Autodesk Inventor part; units mm, degrees
(part 2 of 2)
sketch "Triangle Hole Template x16_1" plane through (0, 0, 0) normal (0, 0, 1) x (1, 0, 0)
  line L0 (-16.6681, -28.8484) -> (-50.0011, -28.8484) construction
  line L1 (-50.0011, -28.8484) -> (-33.3346, 0.0188) construction
  line L2 (-33.3346, 0.0188) -> (-16.6681, -28.8484) construction
  line L3 (-17.5341, -28.3484) -> (-49.1351, -28.3484) construction
  line L4 (-33.3346, -28.8484) -> (-33.3346, -29.3484) construction
  line L5 (-18.5734, -27.7484) -> (-19.2662, -27.3484) construction
  line L6 (-49.1351, -28.3484) -> (-33.3346, -0.9812) construction
  line L7 (-33.3346, -0.9812) -> (-17.5341, -28.3484) construction
  line L8 (-33.3346, -28.3484) -> (-33.3346, -28.8484) construction
  line L9 (-41.2348, -14.6648) -> (-41.6679, -14.4148) construction
  line L10 (-25.4344, -14.6648) -> (-25.0014, -14.4148) construction
  arc A0 (-48.0959, -26.5484) -> (-47.0566, -28.3484) centre (-47.0566, -27.1484) ccw
  arc A1 (-32.2954, -2.7812) -> (-34.3738, -2.7812) centre (-33.3346, -3.3812) ccw
  arc A2 (-19.6126, -28.3484) -> (-18.5734, -26.5484) centre (-19.6126, -27.1484) ccw
  line L11 (-19.6126, -28.3484) -> (-47.0566, -28.3484)
  line L12 (-48.0959, -26.5484) -> (-34.3738, -2.7812)
  line L13 (-32.2954, -2.7812) -> (-18.5734, -26.5484)
  circle A3 centre (-18.227, -27.9484) radius 0.4 construction
  line L14 (-18.5734, -27.7484) -> (-17.8805, -28.1484) construction
  circle A4 centre (-16.6681, -28.8484) radius 3 construction
  line L15 (-49.9979, -28.8484) -> (-16.6649, -28.8484) construction
  line L16 (-16.6649, -28.8484) -> (-33.3314, -57.7156) construction
  line L17 (-33.3314, -57.7156) -> (-49.9979, -28.8484) construction
  line L18 (-49.1319, -29.3484) -> (-17.5309, -29.3484) construction
  line L19 (-33.3314, -28.8484) -> (-33.3314, -28.3484) construction
  line L20 (-48.0926, -29.9484) -> (-47.3998, -30.3484) construction
  line L21 (-17.5309, -29.3484) -> (-33.3314, -56.7156) construction
  line L22 (-33.3314, -56.7156) -> (-49.1319, -29.3484) construction
  line L23 (-33.3314, -29.3484) -> (-33.3314, -28.8484) construction
  line L24 (-25.4312, -43.032) -> (-24.9981, -43.282) construction
  line L25 (-41.2316, -43.032) -> (-41.6646, -43.282) construction
  arc A5 (-18.5701, -31.1484) -> (-19.6094, -29.3484) centre (-19.6094, -30.5484) ccw
  arc A6 (-34.3706, -54.9156) -> (-32.2922, -54.9156) centre (-33.3314, -54.3156) ccw
  arc A7 (-47.0534, -29.3484) -> (-48.0926, -31.1484) centre (-47.0534, -30.5484) ccw
  line L26 (-47.0534, -29.3484) -> (-19.6094, -29.3484)
  line L27 (-18.5701, -31.1484) -> (-32.2922, -54.9156)
  line L28 (-34.3706, -54.9156) -> (-48.0926, -31.1484)
  circle A8 centre (-48.439, -29.7484) radius 0.4 construction
  line L29 (-48.0926, -29.9484) -> (-48.7855, -29.5484) construction
  circle A9 centre (-49.9979, -28.8484) radius 3 construction
  line L30 (-66.6676, 0.0188) -> (-33.3346, 0.0188) construction
  line L31 (-33.3346, 0.0188) -> (-50.0011, -28.8484) construction
  line L32 (-50.0011, -28.8484) -> (-66.6676, 0.0188) construction
  line L33 (-65.8016, -0.4812) -> (-34.2006, -0.4812) construction
  line L34 (-50.0011, 0.0188) -> (-50.0011, 0.5188) construction
  line L35 (-64.7624, -1.0812) -> (-64.0695, -1.4812) construction
  line L36 (-34.2006, -0.4812) -> (-50.0011, -27.8484) construction
  line L37 (-50.0011, -27.8484) -> (-65.8016, -0.4812) construction
  line L38 (-50.0011, -0.4812) -> (-50.0011, 0.0188) construction
  line L39 (-42.1009, -14.1648) -> (-41.6679, -14.4148) construction
  line L40 (-57.9013, -14.1648) -> (-58.3344, -14.4148) construction
  arc A10 (-35.2399, -2.2812) -> (-36.2791, -0.4812) centre (-36.2791, -1.6812) ccw
  arc A11 (-51.0403, -26.0484) -> (-48.9619, -26.0484) centre (-50.0011, -25.4484) ccw
  arc A12 (-63.7231, -0.4812) -> (-64.7624, -2.2812) centre (-63.7231, -1.6812) ccw
  line L41 (-63.7231, -0.4812) -> (-36.2791, -0.4812)
  line L42 (-35.2399, -2.2812) -> (-48.9619, -26.0484)
  line L43 (-51.0403, -26.0484) -> (-64.7624, -2.2812)
  circle A13 centre (-65.1088, -0.8812) radius 0.4 construction
  line L44 (-64.7624, -1.0812) -> (-65.4552, -0.6812) construction
  circle A14 centre (-66.6676, 0.0188) radius 3 construction
  line L45 (-33.3314, 0.0188) -> (0.0016, 0.0188) construction
  line L46 (0.0016, 0.0188) -> (-16.6649, -28.8484) construction
  line L47 (-16.6649, -28.8484) -> (-33.3314, 0.0188) construction
  line L48 (-32.4654, -0.4812) -> (-0.8644, -0.4812) construction
  line L49 (-16.6649, 0.0188) -> (-16.6649, 0.5188) construction
  line L50 (-31.4261, -1.0812) -> (-30.7333, -1.4812) construction
  line L51 (-0.8644, -0.4812) -> (-16.6649, -27.8484) construction
  line L52 (-16.6649, -27.8484) -> (-32.4654, -0.4812) construction
  line L53 (-16.6649, -0.4812) -> (-16.6649, 0.0188) construction
  line L54 (-8.7647, -14.1648) -> (-8.3316, -14.4148) construction
  line L55 (-24.5651, -14.1648) -> (-24.9981, -14.4148) construction
  arc A15 (-1.9036, -2.2812) -> (-2.9429, -0.4812) centre (-2.9429, -1.6812) ccw
  arc A16 (-17.7041, -26.0484) -> (-15.6257, -26.0484) centre (-16.6649, -25.4484) ccw
  arc A17 (-30.3869, -0.4812) -> (-31.4261, -2.2812) centre (-30.3869, -1.6812) ccw
  line L56 (-30.3869, -0.4812) -> (-2.9429, -0.4812)
  line L57 (-1.9036, -2.2812) -> (-15.6257, -26.0484)
  line L58 (-17.7041, -26.0484) -> (-31.4261, -2.2812)
  circle A18 centre (-31.7725, -0.8812) radius 0.4 construction
  line L59 (-31.4261, -1.0812) -> (-32.119, -0.6812) construction
  circle A19 centre (-33.3314, 0.0188) radius 3 construction
  line L60 (-83.317, -28.8188) -> (-49.984, -28.8188) construction
  line L61 (-49.984, -28.8188) -> (-66.6505, -57.686) construction
  line L62 (-66.6505, -57.686) -> (-83.317, -28.8188) construction
  line L63 (-82.451, -29.3188) -> (-50.85, -29.3188) construction
  line L64 (-66.6505, -28.8188) -> (-66.6505, -28.3188) construction
  line L65 (-81.4117, -29.9188) -> (-80.7189, -30.3188) construction
  line L66 (-50.85, -29.3188) -> (-66.6505, -56.686) construction
  line L67 (-66.6505, -56.686) -> (-82.451, -29.3188) construction
  line L68 (-66.6505, -29.3188) -> (-66.6505, -28.8188) construction
  line L69 (-58.7503, -43.0024) -> (-58.3173, -43.2524) construction
  line L70 (-74.5507, -43.0024) -> (-74.9838, -43.2524) construction
  arc A20 (-51.8893, -31.1188) -> (-52.9285, -29.3188) centre (-52.9285, -30.5188) ccw
  arc A21 (-67.6897, -54.886) -> (-65.6113, -54.886) centre (-66.6505, -54.286) ccw
  arc A22 (-80.3725, -29.3188) -> (-81.4117, -31.1188) centre (-80.3725, -30.5188) ccw
  line L71 (-80.3725, -29.3188) -> (-52.9285, -29.3188)
  line L72 (-51.8893, -31.1188) -> (-65.6113, -54.886)
  line L73 (-67.6897, -54.886) -> (-81.4117, -31.1188)
  circle A23 centre (-81.7582, -29.7188) radius 0.4 construction
  line L74 (-81.4117, -29.9188) -> (-82.1046, -29.5188) construction
  circle A24 centre (-83.317, -28.8188) radius 3 construction
  line L75 (-99.9974, 0.0188) -> (-66.6644, 0.0188) construction
  line L76 (-66.6644, 0.0188) -> (-83.3309, -28.8484) construction
  line L77 (-83.3309, -28.8484) -> (-99.9974, 0.0188) construction
  line L78 (-99.1314, -0.4812) -> (-67.5304, -0.4812) construction
  line L79 (-83.3309, 0.0188) -> (-83.3309, 0.5188) construction
  line L80 (-98.0921, -1.0812) -> (-97.3993, -1.4812) construction
  line L81 (-67.5304, -0.4812) -> (-83.3309, -27.8484) construction
  line L82 (-83.3309, -27.8484) -> (-99.1314, -0.4812) construction
  line L83 (-83.3309, -0.4812) -> (-83.3309, 0.0188) construction
  line L84 (-75.4307, -14.1648) -> (-74.9976, -14.4148) construction
  line L85 (-91.2311, -14.1648) -> (-91.6641, -14.4148) construction
  arc A25 (-68.5696, -2.2812) -> (-69.6089, -0.4812) centre (-69.6089, -1.6812) ccw
  arc A26 (-84.3701, -26.0484) -> (-82.2917, -26.0484) centre (-83.3309, -25.4484) ccw
  arc A27 (-97.0529, -0.4812) -> (-98.0921, -2.2812) centre (-97.0529, -1.6812) ccw
  line L86 (-97.0529, -0.4812) -> (-69.6089, -0.4812)
  line L87 (-68.5696, -2.2812) -> (-82.2917, -26.0484)
  line L88 (-84.3701, -26.0484) -> (-98.0921, -2.2812)
  circle A28 centre (-98.4385, -0.8812) radius 0.4 construction
  line L89 (-98.0921, -1.0812) -> (-98.785, -0.6812) construction
  circle A29 centre (-99.9974, 0.0188) radius 3 construction
  line L90 (-133.3304, -0.008) -> (-99.9974, -0.008) construction
  line L91 (-99.9974, -0.008) -> (-116.6639, -28.8752) construction
  line L92 (-116.6639, -28.8752) -> (-133.3304, -0.008) construction
  line L93 (-132.4644, -0.508) -> (-100.8634, -0.508) construction
  line L94 (-116.6639, -0.008) -> (-116.6639, 0.492) construction
  line L95 (-131.4251, -1.108) -> (-130.7323, -1.508) construction
  line L96 (-100.8634, -0.508) -> (-116.6639, -27.8752) construction
  line L97 (-116.6639, -27.8752) -> (-132.4644, -0.508) construction
  line L98 (-116.6639, -0.508) -> (-116.6639, -0.008) construction
  line L99 (-108.7637, -14.1916) -> (-108.3306, -14.4416) construction
  line L100 (-124.5641, -14.1916) -> (-124.9971, -14.4416) construction
  arc A30 (-101.9026, -2.308) -> (-102.9419, -0.508) centre (-102.9419, -1.708) ccw
  arc A31 (-117.7031, -26.0752) -> (-115.6247, -26.0752) centre (-116.6639, -25.4752) ccw
  arc A32 (-130.3859, -0.508) -> (-131.4251, -2.308) centre (-130.3859, -1.708) ccw
  line L101 (-130.3859, -0.508) -> (-102.9419, -0.508)
  line L102 (-101.9026, -2.308) -> (-115.6247, -26.0752)
  line L103 (-117.7031, -26.0752) -> (-131.4251, -2.308)
  circle A33 centre (-131.7715, -0.908) radius 0.4 construction
  line L104 (-131.4251, -1.108) -> (-132.118, -0.708) construction
  circle A34 centre (-133.3304, -0.008) radius 3 construction
  line L105 (-116.6671, -28.8484) -> (-83.3341, -28.8484) construction
  line L106 (-83.3341, -28.8484) -> (-100.0006, -57.7156) construction
  line L107 (-100.0006, -57.7156) -> (-116.6671, -28.8484) construction
  line L108 (-115.8011, -29.3484) -> (-84.2001, -29.3484) construction
  line L109 (-100.0006, -28.8484) -> (-100.0006, -28.3484) construction
  line L110 (-114.7619, -29.9484) -> (-114.069, -30.3484) construction
  line L111 (-84.2001, -29.3484) -> (-100.0006, -56.7156) construction
  line L112 (-100.0006, -56.7156) -> (-115.8011, -29.3484) construction
  line L113 (-100.0006, -29.3484) -> (-100.0006, -28.8484) construction
  line L114 (-92.1004, -43.032) -> (-91.6674, -43.282) construction
  line L115 (-107.9008, -43.032) -> (-108.3339, -43.282) construction
  arc A35 (-85.2394, -31.1484) -> (-86.2786, -29.3484) centre (-86.2786, -30.5484) ccw
  arc A36 (-101.0398, -54.9156) -> (-98.9614, -54.9156) centre (-100.0006, -54.3156) ccw
  arc A37 (-113.7226, -29.3484) -> (-114.7619, -31.1484) centre (-113.7226, -30.5484) ccw
  line L116 (-113.7226, -29.3484) -> (-86.2786, -29.3484)
  line L117 (-85.2394, -31.1484) -> (-98.9614, -54.9156)
  line L118 (-101.0398, -54.9156) -> (-114.7619, -31.1484)
  circle A38 centre (-115.1083, -29.7484) radius 0.4 construction
  line L119 (-114.7619, -29.9484) -> (-115.4547, -29.5484) construction
  circle A39 centre (-116.6671, -28.8484) radius 3 construction
  line L120 (-99.9974, -57.7156) -> (-66.6644, -57.7156) construction
  line L121 (-66.6644, -57.7156) -> (-83.3309, -86.5829) construction
  line L122 (-83.3309, -86.5829) -> (-99.9974, -57.7156) construction
  line L123 (-99.1314, -58.2156) -> (-67.5304, -58.2156) construction
  line L124 (-83.3309, -57.7156) -> (-83.3309, -57.2156) construction
  line L125 (-98.0921, -58.8156) -> (-97.3993, -59.2156) construction
  line L126 (-67.5304, -58.2156) -> (-83.3309, -85.5829) construction
  line L127 (-83.3309, -85.5829) -> (-99.1314, -58.2156) construction
  line L128 (-83.3309, -58.2156) -> (-83.3309, -57.7156) construction
  line L129 (-75.4307, -71.8992) -> (-74.9976, -72.1492) construction
  line L130 (-91.2311, -71.8992) -> (-91.6641, -72.1492) construction
  arc A40 (-68.5696, -60.0156) -> (-69.6089, -58.2156) centre (-69.6089, -59.4156) ccw
  arc A41 (-84.3701, -83.7829) -> (-82.2917, -83.7829) centre (-83.3309, -83.1829) ccw
  arc A42 (-97.0529, -58.2156) -> (-98.0921, -60.0156) centre (-97.0529, -59.4156) ccw
  line L131 (-97.0529, -58.2156) -> (-69.6089, -58.2156)
  line L132 (-68.5696, -60.0156) -> (-82.2917, -83.7829)
  line L133 (-84.3701, -83.7829) -> (-98.0921, -60.0156)
  circle A43 centre (-98.4385, -58.6156) radius 0.4 construction
  line L134 (-98.0921, -58.8156) -> (-98.785, -58.4156) construction
  circle A44 centre (-99.9974, -57.7156) radius 3 construction
  line L135 (-83.3309, -86.5829) -> (-49.9979, -86.5829) construction
  line L136 (-49.9979, -86.5829) -> (-66.6644, -115.4501) construction
  line L137 (-66.6644, -115.4501) -> (-83.3309, -86.5829) construction
  line L138 (-82.4649, -87.0829) -> (-50.8639, -87.0829) construction
  line L139 (-66.6644, -86.5829) -> (-66.6644, -86.0829) construction
  line L140 (-81.4256, -87.6829) -> (-80.7328, -88.0829) construction
  line L141 (-50.8639, -87.0829) -> (-66.6644, -114.4501) construction
  line L142 (-66.6644, -114.4501) -> (-82.4649, -87.0829) construction
  line L143 (-66.6644, -87.0829) -> (-66.6644, -86.5829) construction
  line L144 (-58.7642, -100.7665) -> (-58.3311, -101.0165) construction
  line L145 (-74.5646, -100.7665) -> (-74.9976, -101.0165) construction
  arc A45 (-51.9031, -88.8829) -> (-52.9424, -87.0829) centre (-52.9424, -88.2829) ccw
  arc A46 (-67.7036, -112.6501) -> (-65.6252, -112.6501) centre (-66.6644, -112.0501) ccw
  arc A47 (-80.3864, -87.0829) -> (-81.4256, -88.8829) centre (-80.3864, -88.2829) ccw
  line L146 (-80.3864, -87.0829) -> (-52.9424, -87.0829)
  line L147 (-51.9031, -88.8829) -> (-65.6252, -112.6501)
  line L148 (-67.7036, -112.6501) -> (-81.4256, -88.8829)
  circle A48 centre (-81.772, -87.4829) radius 0.4 construction
  line L149 (-81.4256, -87.6829) -> (-82.1185, -87.2829) construction
  circle A49 centre (-83.3309, -86.5829) radius 3 construction
  line L150 (-66.6676, -57.7533) -> (-33.3346, -57.7533) construction
  line L151 (-33.3346, -57.7533) -> (-50.0011, -86.6205) construction
  line L152 (-50.0011, -86.6205) -> (-66.6676, -57.7533) construction
  line L153 (-65.8016, -58.2533) -> (-34.2006, -58.2533) construction
  line L154 (-50.0011, -57.7533) -> (-50.0011, -57.2533) construction
  line L155 (-64.7624, -58.8533) -> (-64.0695, -59.2533) construction
  line L156 (-34.2006, -58.2533) -> (-50.0011, -85.6205) construction
  line L157 (-50.0011, -85.6205) -> (-65.8016, -58.2533) construction
  line L158 (-50.0011, -58.2533) -> (-50.0011, -57.7533) construction
  line L159 (-42.1009, -71.9369) -> (-41.6679, -72.1869) construction
  line L160 (-57.9013, -71.9369) -> (-58.3344, -72.1869) construction
  arc A50 (-35.2399, -60.0533) -> (-36.2791, -58.2533) centre (-36.2791, -59.4533) ccw
  arc A51 (-51.0403, -83.8205) -> (-48.9619, -83.8205) centre (-50.0011, -83.2205) ccw
  arc A52 (-63.7231, -58.2533) -> (-64.7624, -60.0533) centre (-63.7231, -59.4533) ccw
  line L161 (-63.7231, -58.2533) -> (-36.2791, -58.2533)
  line L162 (-35.2399, -60.0533) -> (-48.9619, -83.8205)
  line L163 (-51.0403, -83.8205) -> (-64.7624, -60.0533)
  circle A53 centre (-65.1088, -58.6533) radius 0.4 construction
  line L164 (-64.7624, -58.8533) -> (-65.4552, -58.4533) construction
  circle A54 centre (-66.6676, -57.7533) radius 3 construction
  line L165 (-50.0011, -86.6205) -> (-83.3341, -86.6205) construction
  line L166 (-83.3341, -86.6205) -> (-66.6676, -57.7533) construction
  line L167 (-66.6676, -57.7533) -> (-50.0011, -86.6205) construction
  line L168 (-50.8671, -86.1205) -> (-82.4681, -86.1205) construction
  line L169 (-66.6676, -86.6205) -> (-66.6676, -87.1205) construction
  line L170 (-51.9064, -85.5205) -> (-52.5992, -85.1205) construction
  line L171 (-82.4681, -86.1205) -> (-66.6676, -58.7533) construction
  line L172 (-66.6676, -58.7533) -> (-50.8671, -86.1205) construction
  line L173 (-66.6676, -86.1205) -> (-66.6676, -86.6205) construction
  line L174 (-74.5678, -72.4369) -> (-75.0009, -72.1869) construction
  line L175 (-58.7674, -72.4369) -> (-58.3344, -72.1869) construction
  arc A55 (-81.4289, -84.3205) -> (-80.3896, -86.1205) centre (-80.3896, -84.9205) ccw
  arc A56 (-65.6284, -60.5533) -> (-67.7068, -60.5533) centre (-66.6676, -61.1533) ccw
  arc A57 (-52.9456, -86.1205) -> (-51.9064, -84.3205) centre (-52.9456, -84.9205) ccw
  line L176 (-52.9456, -86.1205) -> (-80.3896, -86.1205)
  line L177 (-81.4289, -84.3205) -> (-67.7068, -60.5533)
  line L178 (-65.6284, -60.5533) -> (-51.9064, -84.3205)
  circle A58 centre (-51.56, -85.7205) radius 0.4 construction
  line L179 (-51.9064, -85.5205) -> (-51.2135, -85.9205) construction
  circle A59 centre (-50.0011, -86.6205) radius 3 construction
  line L180 (-33.3346, -57.7533) -> (-66.6676, -57.7533) construction
  line L181 (-66.6676, -57.7533) -> (-50.0011, -28.886) construction
  line L182 (-50.0011, -28.886) -> (-33.3346, -57.7533) construction
  line L183 (-34.2006, -57.2533) -> (-65.8016, -57.2533) construction
  line L184 (-50.0011, -57.7533) -> (-50.0011, -58.2533) construction
  line L185 (-35.2399, -56.6533) -> (-35.9327, -56.2533) construction
  line L186 (-65.8016, -57.2533) -> (-50.0011, -29.886) construction
  line L187 (-50.0011, -29.886) -> (-34.2006, -57.2533) construction
  line L188 (-50.0011, -57.2533) -> (-50.0011, -57.7533) construction
  line L189 (-57.9013, -43.5697) -> (-58.3344, -43.3197) construction
  line L190 (-42.1009, -43.5697) -> (-41.6679, -43.3197) construction
  arc A60 (-64.7624, -55.4533) -> (-63.7231, -57.2533) centre (-63.7231, -56.0533) ccw
  arc A61 (-48.9619, -31.686) -> (-51.0403, -31.686) centre (-50.0011, -32.286) ccw
  arc A62 (-36.2791, -57.2533) -> (-35.2399, -55.4533) centre (-36.2791, -56.0533) ccw
  line L191 (-36.2791, -57.2533) -> (-63.7231, -57.2533)
  line L192 (-64.7624, -55.4533) -> (-51.0403, -31.686)
  line L193 (-48.9619, -31.686) -> (-35.2399, -55.4533)
  circle A63 centre (-34.8935, -56.8533) radius 0.4 construction
  line L194 (-35.2399, -56.6533) -> (-34.547, -57.0533) construction
  circle A64 centre (-33.3346, -57.7533) radius 3 construction
  line L195 (-66.6676, -57.7156) -> (-100.0006, -57.7156) construction
  line L196 (-100.0006, -57.7156) -> (-83.3341, -28.8484) construction
  line L197 (-83.3341, -28.8484) -> (-66.6676, -57.7156) construction
  line L198 (-67.5336, -57.2156) -> (-99.1346, -57.2156) construction
  line L199 (-83.3341, -57.7156) -> (-83.3341, -58.2156) construction
  line L200 (-68.5729, -56.6156) -> (-69.2657, -56.2156) construction
  line L201 (-99.1346, -57.2156) -> (-83.3341, -29.8484) construction
  line L202 (-83.3341, -29.8484) -> (-67.5336, -57.2156) construction
  line L203 (-83.3341, -57.2156) -> (-83.3341, -57.7156) construction
  line L204 (-91.2343, -43.532) -> (-91.6674, -43.282) construction
  line L205 (-75.4339, -43.532) -> (-75.0009, -43.282) construction
  arc A65 (-98.0954, -55.4156) -> (-97.0561, -57.2156) centre (-97.0561, -56.0156) ccw
  arc A66 (-82.2949, -31.6484) -> (-84.3733, -31.6484) centre (-83.3341, -32.2484) ccw
  arc A67 (-69.6121, -57.2156) -> (-68.5729, -55.4156) centre (-69.6121, -56.0156) ccw
  line L206 (-69.6121, -57.2156) -> (-97.0561, -57.2156)
  line L207 (-98.0954, -55.4156) -> (-84.3733, -31.6484)
  line L208 (-82.2949, -31.6484) -> (-68.5729, -55.4156)
  circle A68 centre (-68.2265, -56.8156) radius 0.4 construction
  line L209 (-68.5729, -56.6156) -> (-67.88, -57.0156) construction
  circle A69 centre (-66.6676, -57.7156) radius 3 construction
  line L210 (-83.3186, -28.8752) -> (-116.6516, -28.8752) construction
  line L211 (-116.6516, -28.8752) -> (-99.9851, -0.008) construction
  line L212 (-99.9851, -0.008) -> (-83.3186, -28.8752) construction
  line L213 (-84.1846, -28.3752) -> (-115.7856, -28.3752) construction
  line L214 (-99.9851, -28.8752) -> (-99.9851, -29.3752) construction
  line L215 (-85.2239, -27.7752) -> (-85.9167, -27.3752) construction
  line L216 (-115.7856, -28.3752) -> (-99.9851, -1.008) construction
  line L217 (-99.9851, -1.008) -> (-84.1846, -28.3752) construction
  line L218 (-99.9851, -28.3752) -> (-99.9851, -28.8752) construction
  line L219 (-107.8853, -14.6916) -> (-108.3184, -14.4416) construction
  line L220 (-92.0849, -14.6916) -> (-91.6519, -14.4416) construction
  arc A70 (-114.7464, -26.5752) -> (-113.7071, -28.3752) centre (-113.7071, -27.1752) ccw
  arc A71 (-98.9459, -2.808) -> (-101.0243, -2.808) centre (-99.9851, -3.408) ccw
  arc A72 (-86.2631, -28.3752) -> (-85.2239, -26.5752) centre (-86.2631, -27.1752) ccw
  line L221 (-86.2631, -28.3752) -> (-113.7071, -28.3752)
  line L222 (-114.7464, -26.5752) -> (-101.0243, -2.808)
  line L223 (-98.9459, -2.808) -> (-85.2239, -26.5752)
  circle A73 centre (-84.8775, -27.9752) radius 0.4 construction
  line L224 (-85.2239, -27.7752) -> (-84.531, -28.1752) construction
  circle A74 centre (-83.3186, -28.8752) radius 3 construction
  line L225 (-50.0011, -28.8484) -> (-83.3341, -28.8484) construction
  line L226 (-83.3341, -28.8484) -> (-66.6676, 0.0188) construction
  line L227 (-66.6676, 0.0188) -> (-50.0011, -28.8484) construction
  line L228 (-50.8671, -28.3484) -> (-82.4681, -28.3484) construction
  line L229 (-66.6676, -28.8484) -> (-66.6676, -29.3484) construction
  line L230 (-51.9064, -27.7484) -> (-52.5992, -27.3484) construction
  line L231 (-82.4681, -28.3484) -> (-66.6676, -0.9812) construction
  line L232 (-66.6676, -0.9812) -> (-50.8671, -28.3484) construction
  line L233 (-66.6676, -28.3484) -> (-66.6676, -28.8484) construction
  line L234 (-74.5678, -14.6648) -> (-75.0009, -14.4148) construction
  line L235 (-58.7674, -14.6648) -> (-58.3344, -14.4148) construction
  arc A75 (-81.4289, -26.5484) -> (-80.3896, -28.3484) centre (-80.3896, -27.1484) ccw
  arc A76 (-65.6284, -2.7812) -> (-67.7068, -2.7812) centre (-66.6676, -3.3812) ccw
  arc A77 (-52.9456, -28.3484) -> (-51.9064, -26.5484) centre (-52.9456, -27.1484) ccw
  line L236 (-52.9456, -28.3484) -> (-80.3896, -28.3484)
  line L237 (-81.4289, -26.5484) -> (-67.7068, -2.7812)
  line L238 (-65.6284, -2.7812) -> (-51.9064, -26.5484)
  circle A78 centre (-51.56, -27.9484) radius 0.4 construction
  line L239 (-51.9064, -27.7484) -> (-51.2135, -28.1484) construction
  circle A79 centre (-50.0011, -28.8484) radius 3 construction
  point P0 (-67.2349, -38.1612)
derived "g16-ledbase.ipt"
sketch "Strut Templates" plane through (0, 0, 0) normal (0, 1, 0) x (-1, 0, 0)
  circle A0 centre (16.6665, 28.8672) radius 1.5
  circle A1 centre (33.333, 57.7344) radius 1.5
  circle A2 centre (0, 0) radius 1.5
  circle A3 centre (33.333, 0) radius 1.5
  circle A4 centre (66.666, 0) radius 1.5
  circle A5 centre (99.999, 0) radius 1.5
  circle A6 centre (133.332, 0) radius 1.5
  circle A7 centre (116.6655, 28.8672) radius 1.5
  circle A8 centre (99.999, 57.7344) radius 1.5
  circle A9 centre (83.3325, 86.6017) radius 1.5
  circle A10 centre (49.9995, 86.6017) radius 1.5
  circle A11 centre (66.666, 115.4689) radius 1.5
  arc A12 (-2.5981, 1.5) -> (0, -3) centre (0, 0) ccw
  line L0 (0, -3) -> (133.332, -3)
  arc A13 (36.333, 0) -> (30.333, 0) centre (33.333, 0) ccw
  circle A14 centre (49.9995, 86.6017) radius 3 construction
  line L1 (-2.5981, 1.5) -> (57.2344, 105.1329)
  circle A15 centre (16.6665, 28.8672) radius 3 construction
  circle A16 centre (33.333, 57.7344) radius 3 construction
  line L2 (29.333, -1) -> (4, -1)
  arc A17 (29.333, -1) -> (30.333, 0) centre (29.333, 0) ccw
  circle A18 centre (0, 0) radius 3 construction
  arc A19 (3, 0) -> (1.5, 2.5981) centre (0, 0) ccw
  arc A20 (3, 0) -> (4, -1) centre (4, 0) ccw
  arc A21 (1.134, 3.9641) -> (1.5, 2.5981) centre (2, 3.4641) ccw
  line L3 (1.134, 3.9641) -> (13.8005, 25.9031)
  arc A22 (15.1665, 26.2691) -> (13.8005, 25.9031) centre (14.6665, 25.4031) ccw
  arc A23 (15.1665, 26.2691) -> (18.1665, 31.4653) centre (16.6665, 28.8672) ccw
  arc A24 (17.8005, 32.8313) -> (18.1665, 31.4653) centre (18.6665, 32.3313) ccw
  line L4 (17.8005, 32.8313) -> (30.467, 54.7703)
  line L5 (34.467, 61.6986) -> (47.1335, 83.6376)
  arc A25 (31.833, 55.1364) -> (30.467, 54.7703) centre (31.333, 54.2703) ccw
  arc A26 (31.833, 55.1364) -> (34.833, 60.3325) centre (33.333, 57.7344) ccw
  arc A27 (34.467, 61.6986) -> (34.833, 60.3325) centre (35.333, 61.1986) ccw
  arc A28 (48.4995, 84.0036) -> (51.4995, 89.1998) centre (49.9995, 86.6017) ccw
  arc A29 (51.1335, 90.5658) -> (51.4995, 89.1998) centre (51.9995, 90.0658) ccw
  arc A30 (48.4995, 84.0036) -> (47.1335, 83.6376) centre (47.9995, 83.1376) ccw
  arc A31 (69.2641, 116.9689) -> (64.0679, 116.9689) centre (66.666, 115.4689) ccw
  line L6 (64.0679, 116.9689) -> (57.235, 105.1339)
  line L7 (51.1335, 90.5658) -> (57.9664, 102.4008)
  line L8 (57.235, 105.1339) -> (57.967, 102.4018)
  line L9 (57.967, 102.4018) -> (63.8, 112.5048)
  line L10 (57.9664, 102.4008) -> (57.2344, 105.1329)
  arc A32 (65.166, 112.8708) -> (68.166, 112.8708) centre (66.666, 115.4689) ccw
  arc A33 (65.166, 112.8708) -> (63.8, 112.5048) centre (64.666, 112.0048) ccw
  arc A34 (133.332, -3) -> (130.332, 0) centre (133.332, 0) ccw
  line L11 (69.2641, 116.9689) -> (119.2636, 30.3672)
  arc A35 (102.999, 0) -> (96.999, 0) centre (99.999, 0) ccw
  arc A36 (115.1655, 31.4653) -> (119.2636, 30.3672) centre (116.6655, 28.8672) ccw
  arc A37 (98.499, 60.3325) -> (101.499, 55.1364) centre (99.999, 57.7344) ccw
  arc A38 (81.8325, 89.1998) -> (84.8325, 84.0036) centre (83.3325, 86.6017) ccw
  line L12 (70.666, -1) -> (95.999, -1)
  line L13 (103.999, -1) -> (129.332, -1)
  line L14 (115.5315, 32.8313) -> (102.865, 54.7703)
  line L15 (98.865, 61.6986) -> (86.1985, 83.6376)
  line L16 (82.1985, 90.5658) -> (69.532, 112.5048)
  arc A39 (69.666, 0) -> (70.666, -1) centre (70.666, 0) ccw
  arc A40 (95.999, -1) -> (96.999, 0) centre (95.999, 0) ccw
  arc A41 (102.999, 0) -> (103.999, -1) centre (103.999, 0) ccw
  arc A42 (129.332, -1) -> (130.332, 0) centre (129.332, 0) ccw
  arc A43 (69.532, 112.5048) -> (68.166, 112.8708) centre (68.666, 112.0048) ccw
  arc A44 (81.8325, 89.1998) -> (82.1985, 90.5658) centre (81.3325, 90.0658) ccw
  arc A45 (86.1985, 83.6376) -> (84.8325, 84.0036) centre (85.3325, 83.1376) ccw
  arc A46 (98.499, 60.3325) -> (98.865, 61.6986) centre (97.999, 61.1986) ccw
  arc A47 (102.865, 54.7703) -> (101.499, 55.1364) centre (101.999, 54.2703) ccw
  arc A48 (115.1655, 31.4653) -> (115.5315, 32.8313) centre (114.6655, 32.3313) ccw
  line L17 (37.333, -1) -> (62.666, -1)
  arc A49 (36.333, 0) -> (37.333, -1) centre (37.333, 0) ccw
  arc A50 (62.666, -1) -> (63.666, 0) centre (62.666, 0) ccw
  arc A51 (69.666, 0) -> (63.666, 0) centre (66.666, 0) ccw
  line L18 (0, 0) -> (133.332, 0) construction
  line L19 (16.6665, 28.8672) -> (116.6655, 28.8672) construction
  line L20 (49.9995, 86.6017) -> (83.3325, 86.6017) construction
  line L21 (16.6665, 28.8672) -> (16.6665, 0) construction
  line L22 (33.333, 57.7344) -> (99.999, 57.7344) construction
  line L23 (33.333, 57.7344) -> (33.333, 28.8672) construction
  line L24 (49.9995, 86.6017) -> (49.9995, 57.7344) construction
  line L25 (66.666, 115.4689) -> (66.666, 86.6017) construction
  line L26 (83.3325, 86.6017) -> (83.3325, 0) construction
  line L27 (116.6655, 28.8672) -> (116.6655, 0) construction
  line L28 (99.999, 57.7344) -> (99.999, 0) construction
  line L29 (66.666, 86.6017) -> (66.666, 0) construction
  line L30 (49.9995, 57.7344) -> (49.9995, 0) construction
  line L31 (33.333, 28.8672) -> (33.333, 0) construction
  line L32 (8.3333, 19.5586) -> (24.9998, 19.5586) construction
  line L33 (24.9998, 19.5586) -> (24.9998, 9.3086) construction
  line L34 (24.9998, 9.3086) -> (8.3333, 9.3086) construction
  line L35 (8.3333, 9.3086) -> (8.3333, 19.5586) construction
  line L36 (14.1665, 16.9336) -> (19.1665, 16.9336) construction
  line L37 (19.1665, 16.9336) -> (19.1665, 11.9336) construction
  line L38 (19.1665, 11.9336) -> (14.1665, 11.9336) construction
  line L39 (14.1665, 11.9336) -> (14.1665, 16.9336) construction
  line L40 (16.6665, 19.5586) -> (16.6665, 9.3086) construction
  line L41 (8.3333, 14.4336) -> (24.9998, 14.4336) construction
  line L42 (19.6665, 17.4336) -> (22.1665, 17.4336) construction
  line L43 (22.1665, 17.4336) -> (22.1665, 11.4336) construction
  line L44 (22.1665, 11.4336) -> (19.6665, 11.4336) construction
  line L45 (19.6665, 11.4336) -> (19.6665, 17.4336) construction
  line L46 (12.1665, 9.3086) -> (12.1665, 19.5586) construction
  line L47 (24.1665, 9.3086) -> (24.1665, 19.5586) construction
  line L48 (24.9998, 19.5586) -> (41.6663, 19.5586) construction
  line L49 (41.6663, 19.5586) -> (41.6663, 9.3086) construction
  line L50 (41.6663, 9.3086) -> (24.9998, 9.3086) construction
  line L51 (24.9998, 9.3086) -> (24.9998, 19.5586) construction
  line L52 (30.833, 16.9336) -> (35.833, 16.9336) construction
  line L53 (35.833, 16.9336) -> (35.833, 11.9336) construction
  line L54 (35.833, 11.9336) -> (30.833, 11.9336) construction
  line L55 (30.833, 11.9336) -> (30.833, 16.9336) construction
  line L56 (33.333, 19.5586) -> (33.333, 9.3086) construction
  line L57 (24.9998, 14.4336) -> (41.6663, 14.4336) construction
  line L58 (36.333, 17.4336) -> (38.833, 17.4336) construction
  line L59 (38.833, 17.4336) -> (38.833, 11.4336) construction
  line L60 (38.833, 11.4336) -> (36.333, 11.4336) construction
  line L61 (36.333, 11.4336) -> (36.333, 17.4336) construction
  line L62 (28.833, 9.3086) -> (28.833, 19.5586) construction
  line L63 (40.833, 9.3086) -> (40.833, 19.5586) construction
  line L64 (41.6663, 19.5586) -> (58.3328, 19.5586) construction
  line L65 (58.3328, 19.5586) -> (58.3328, 9.3086) construction
  line L66 (58.3328, 9.3086) -> (41.6663, 9.3086) construction
  line L67 (41.6663, 9.3086) -> (41.6663, 19.5586) construction
  line L68 (47.4995, 16.9336) -> (52.4995, 16.9336) construction
  line L69 (52.4995, 16.9336) -> (52.4995, 11.9336) construction
  line L70 (52.4995, 11.9336) -> (47.4995, 11.9336) construction
  line L71 (47.4995, 11.9336) -> (47.4995, 16.9336) construction
  line L72 (49.9995, 19.5586) -> (49.9995, 9.3086) construction
  line L73 (41.6663, 14.4336) -> (58.3328, 14.4336) construction
  line L74 (52.9995, 17.4336) -> (55.4995, 17.4336) construction
  line L75 (55.4995, 17.4336) -> (55.4995, 11.4336) construction
  line L76 (55.4995, 11.4336) -> (52.9995, 11.4336) construction
  line L77 (52.9995, 11.4336) -> (52.9995, 17.4336) construction
  line L78 (45.4995, 9.3086) -> (45.4995, 19.5586) construction
  line L79 (57.4995, 9.3086) -> (57.4995, 19.5586) construction
  line L80 (58.3328, 19.5586) -> (74.9993, 19.5586) construction
  line L81 (74.9993, 19.5586) -> (74.9993, 9.3086) construction
  line L82 (74.9993, 9.3086) -> (58.3328, 9.3086) construction
  line L83 (58.3328, 9.3086) -> (58.3328, 19.5586) construction
  line L84 (64.166, 16.9336) -> (69.166, 16.9336) construction
  line L85 (69.166, 16.9336) -> (69.166, 11.9336) construction
  line L86 (69.166, 11.9336) -> (64.166, 11.9336) construction
  line L87 (64.166, 11.9336) -> (64.166, 16.9336) construction
  line L88 (66.666, 19.5586) -> (66.666, 9.3086) construction
  line L89 (58.3328, 14.4336) -> (74.9993, 14.4336) construction
  line L90 (69.666, 17.4336) -> (72.166, 17.4336) construction
  line L91 (72.166, 17.4336) -> (72.166, 11.4336) construction
  line L92 (72.166, 11.4336) -> (69.666, 11.4336) construction
  line L93 (69.666, 11.4336) -> (69.666, 17.4336) construction
  line L94 (62.166, 9.3086) -> (62.166, 19.5586) construction
  line L95 (74.166, 9.3086) -> (74.166, 19.5586) construction
  line L96 (91.6658, 19.5586) -> (108.3323, 19.5586) construction
  line L97 (108.3323, 19.5586) -> (108.3323, 9.3086) construction
  line L98 (108.3323, 9.3086) -> (91.6658, 9.3086) construction
  line L99 (91.6658, 9.3086) -> (91.6658, 19.5586) construction
  line L100 (97.499, 16.9336) -> (102.499, 16.9336) construction
  line L101 (102.499, 16.9336) -> (102.499, 11.9336) construction
  line L102 (102.499, 11.9336) -> (97.499, 11.9336) construction
  line L103 (97.499, 11.9336) -> (97.499, 16.9336) construction
  line L104 (99.999, 19.5586) -> (99.999, 9.3086) construction
  line L105 (91.6658, 14.4336) -> (108.3323, 14.4336) construction
  line L106 (102.999, 17.4336) -> (105.499, 17.4336) construction
  line L107 (105.499, 17.4336) -> (105.499, 11.4336) construction
  line L108 (105.499, 11.4336) -> (102.999, 11.4336) construction
  line L109 (102.999, 11.4336) -> (102.999, 17.4336) construction
  line L110 (95.499, 9.3086) -> (95.499, 19.5586) construction
  line L111 (107.499, 9.3086) -> (107.499, 19.5586) construction
  line L112 (74.9993, 19.5586) -> (91.6658, 19.5586) construction
  line L113 (91.6658, 19.5586) -> (91.6658, 9.3086) construction
  line L114 (91.6658, 9.3086) -> (74.9993, 9.3086) construction
  line L115 (74.9993, 9.3086) -> (74.9993, 19.5586) construction
  line L116 (80.8325, 16.9336) -> (85.8325, 16.9336) construction
  line L117 (85.8325, 16.9336) -> (85.8325, 11.9336) construction
  line L118 (85.8325, 11.9336) -> (80.8325, 11.9336) construction
  line L119 (80.8325, 11.9336) -> (80.8325, 16.9336) construction
  line L120 (83.3325, 19.5586) -> (83.3325, 9.3086) construction
  line L121 (74.9993, 14.4336) -> (91.6658, 14.4336) construction
  line L122 (86.3325, 17.4336) -> (88.8325, 17.4336) construction
  line L123 (88.8325, 17.4336) -> (88.8325, 11.4336) construction
  line L124 (88.8325, 11.4336) -> (86.3325, 11.4336) construction
  line L125 (86.3325, 11.4336) -> (86.3325, 17.4336) construction
  line L126 (78.8325, 9.3086) -> (78.8325, 19.5586) construction
  line L127 (90.8325, 9.3086) -> (90.8325, 19.5586) construction
  line L128 (108.3323, 19.5586) -> (124.9988, 19.5586) construction
  line L129 (124.9988, 19.5586) -> (124.9988, 9.3086) construction
  line L130 (124.9988, 9.3086) -> (108.3323, 9.3086) construction
  line L131 (108.3323, 9.3086) -> (108.3323, 19.5586) construction
  line L132 (114.1655, 16.9336) -> (119.1655, 16.9336) construction
  line L133 (119.1655, 16.9336) -> (119.1655, 11.9336) construction
  line L134 (119.1655, 11.9336) -> (114.1655, 11.9336) construction
  line L135 (114.1655, 11.9336) -> (114.1655, 16.9336) construction
  line L136 (116.6655, 19.5586) -> (116.6655, 9.3086) construction
  line L137 (108.3323, 14.4336) -> (124.9988, 14.4336) construction
  line L138 (119.6655, 17.4336) -> (122.1655, 17.4336) construction
  line L139 (122.1655, 17.4336) -> (122.1655, 11.4336) construction
  line L140 (122.1655, 11.4336) -> (119.6655, 11.4336) construction
  line L141 (119.6655, 11.4336) -> (119.6655, 17.4336) construction
  line L142 (112.1655, 9.3086) -> (112.1655, 19.5586) construction
  line L143 (124.1655, 9.3086) -> (124.1655, 19.5586) construction
  line L144 (58.3328, 77.2931) -> (74.9993, 77.2931) construction
  line L145 (74.9993, 77.2931) -> (74.9993, 67.0431) construction
  line L146 (74.9993, 67.0431) -> (58.3328, 67.0431) construction
  line L147 (58.3328, 67.0431) -> (58.3328, 77.2931) construction
  line L148 (64.166, 74.6681) -> (69.166, 74.6681) construction
  line L149 (69.166, 74.6681) -> (69.166, 69.6681) construction
  line L150 (69.166, 69.6681) -> (64.166, 69.6681) construction
  line L151 (64.166, 69.6681) -> (64.166, 74.6681) construction
  line L152 (66.666, 77.2931) -> (66.666, 67.0431) construction
  line L153 (58.3328, 72.1681) -> (74.9993, 72.1681) construction
  line L154 (69.666, 75.1681) -> (72.166, 75.1681) construction
  line L155 (72.166, 75.1681) -> (72.166, 69.1681) construction
  line L156 (72.166, 69.1681) -> (69.666, 69.1681) construction
  line L157 (69.666, 69.1681) -> (69.666, 75.1681) construction
  line L158 (62.166, 67.0431) -> (62.166, 77.2931) construction
  line L159 (74.166, 67.0431) -> (74.166, 77.2931) construction
  line L160 (74.9993, 77.2931) -> (91.6658, 77.2931) construction
  line L161 (91.6658, 77.2931) -> (91.6658, 67.0431) construction
  line L162 (91.6658, 67.0431) -> (74.9993, 67.0431) construction
  line L163 (74.9993, 67.0431) -> (74.9993, 77.2931) construction
  line L164 (80.8325, 74.6681) -> (85.8325, 74.6681) construction
  line L165 (85.8325, 74.6681) -> (85.8325, 69.6681) construction
  line L166 (85.8325, 69.6681) -> (80.8325, 69.6681) construction
  line L167 (80.8325, 69.6681) -> (80.8325, 74.6681) construction
  line L168 (83.3325, 77.2931) -> (83.3325, 67.0431) construction
  line L169 (74.9993, 72.1681) -> (91.6658, 72.1681) construction
  line L170 (86.3325, 75.1681) -> (88.8325, 75.1681) construction
  line L171 (88.8325, 75.1681) -> (88.8325, 69.1681) construction
  line L172 (88.8325, 69.1681) -> (86.3325, 69.1681) construction
  line L173 (86.3325, 69.1681) -> (86.3325, 75.1681) construction
  line L174 (78.8325, 67.0431) -> (78.8325, 77.2931) construction
  line L175 (90.8325, 67.0431) -> (90.8325, 77.2931) construction
  line L176 (108.3323, 38.1758) -> (91.6658, 38.1758) construction
  line L177 (91.6658, 38.1758) -> (91.6658, 48.4258) construction
  line L178 (91.6658, 48.4258) -> (108.3323, 48.4258) construction
  line L179 (108.3323, 48.4258) -> (108.3323, 38.1758) construction
  line L180 (102.499, 40.8008) -> (97.499, 40.8008) construction
  line L181 (97.499, 40.8008) -> (97.499, 45.8008) construction
  line L182 (97.499, 45.8008) -> (102.499, 45.8008) construction
  line L183 (102.499, 45.8008) -> (102.499, 40.8008) construction
  line L184 (99.999, 38.1758) -> (99.999, 48.4258) construction
  line L185 (108.3323, 43.3008) -> (91.6658, 43.3008) construction
  line L186 (96.999, 40.3008) -> (94.499, 40.3008) construction
  line L187 (94.499, 40.3008) -> (94.499, 46.3008) construction
  line L188 (94.499, 46.3008) -> (96.999, 46.3008) construction
  line L189 (96.999, 46.3008) -> (96.999, 40.3008) construction
  line L190 (104.499, 48.4258) -> (104.499, 38.1758) construction
  line L191 (92.499, 48.4258) -> (92.499, 38.1758) construction
  line L192 (41.6663, 77.2931) -> (58.3328, 77.2931) construction
  line L193 (58.3328, 77.2931) -> (58.3328, 67.0431) construction
  line L194 (58.3328, 67.0431) -> (41.6663, 67.0431) construction
  line L195 (41.6663, 67.0431) -> (41.6663, 77.2931) construction
  line L196 (47.4995, 74.6681) -> (52.4995, 74.6681) construction
  line L197 (52.4995, 74.6681) -> (52.4995, 69.6681) construction
  line L198 (52.4995, 69.6681) -> (47.4995, 69.6681) construction
  line L199 (47.4995, 69.6681) -> (47.4995, 74.6681) construction
  line L200 (49.9995, 77.2931) -> (49.9995, 67.0431) construction
  line L201 (41.6663, 72.1681) -> (58.3328, 72.1681) construction
  line L202 (52.9995, 75.1681) -> (55.4995, 75.1681) construction
  line L203 (55.4995, 75.1681) -> (55.4995, 69.1681) construction
  line L204 (55.4995, 69.1681) -> (52.9995, 69.1681) construction
  line L205 (52.9995, 69.1681) -> (52.9995, 75.1681) construction
  line L206 (45.4995, 67.0431) -> (45.4995, 77.2931) construction
  line L207 (57.4995, 67.0431) -> (57.4995, 77.2931) construction
  line L208 (74.9993, 38.1758) -> (58.3328, 38.1758) construction
  line L209 (58.3328, 38.1758) -> (58.3328, 48.4258) construction
  line L210 (58.3328, 48.4258) -> (74.9993, 48.4258) construction
  line L211 (74.9993, 48.4258) -> (74.9993, 38.1758) construction
  line L212 (69.166, 40.8008) -> (64.166, 40.8008) construction
  line L213 (64.166, 40.8008) -> (64.166, 45.8008) construction
  line L214 (64.166, 45.8008) -> (69.166, 45.8008) construction
  line L215 (69.166, 45.8008) -> (69.166, 40.8008) construction
  line L216 (66.666, 38.1758) -> (66.666, 48.4258) construction
  line L217 (74.9993, 43.3008) -> (58.3328, 43.3008) construction
  line L218 (63.666, 40.3008) -> (61.166, 40.3008) construction
  line L219 (61.166, 40.3008) -> (61.166, 46.3008) construction
  line L220 (61.166, 46.3008) -> (63.666, 46.3008) construction
  line L221 (63.666, 46.3008) -> (63.666, 40.3008) construction
  line L222 (71.166, 48.4258) -> (71.166, 38.1758) construction
  line L223 (59.166, 48.4258) -> (59.166, 38.1758) construction
  line L224 (58.3328, 38.1758) -> (41.6663, 38.1758) construction
  line L225 (41.6663, 38.1758) -> (41.6663, 48.4258) construction
  line L226 (41.6663, 48.4258) -> (58.3328, 48.4258) construction
  line L227 (58.3328, 48.4258) -> (58.3328, 38.1758) construction
  line L228 (52.4995, 40.8008) -> (47.4995, 40.8008) construction
  line L229 (47.4995, 40.8008) -> (47.4995, 45.8008) construction
  line L230 (47.4995, 45.8008) -> (52.4995, 45.8008) construction
  line L231 (52.4995, 45.8008) -> (52.4995, 40.8008) construction
  line L232 (49.9995, 38.1758) -> (49.9995, 48.4258) construction
  line L233 (58.3328, 43.3008) -> (41.6663, 43.3008) construction
  line L234 (46.9995, 40.3008) -> (44.4995, 40.3008) construction
  line L235 (44.4995, 40.3008) -> (44.4995, 46.3008) construction
  line L236 (44.4995, 46.3008) -> (46.9995, 46.3008) construction
  line L237 (46.9995, 46.3008) -> (46.9995, 40.3008) construction
  line L238 (54.4995, 48.4258) -> (54.4995, 38.1758) construction
  line L239 (42.4995, 48.4258) -> (42.4995, 38.1758) construction
  line L240 (91.6658, 38.1758) -> (74.9993, 38.1758) construction
  line L241 (74.9993, 38.1758) -> (74.9993, 48.4258) construction
  line L242 (74.9993, 48.4258) -> (91.6658, 48.4258) construction
  line L243 (91.6658, 48.4258) -> (91.6658, 38.1758) construction
  line L244 (85.8325, 40.8008) -> (80.8325, 40.8008) construction
  line L245 (80.8325, 40.8008) -> (80.8325, 45.8008) construction
  line L246 (80.8325, 45.8008) -> (85.8325, 45.8008) construction
  line L247 (85.8325, 45.8008) -> (85.8325, 40.8008) construction
  line L248 (83.3325, 38.1758) -> (83.3325, 48.4258) construction
  line L249 (91.6658, 43.3008) -> (74.9993, 43.3008) construction
  line L250 (80.3325, 40.3008) -> (77.8325, 40.3008) construction
  line L251 (77.8325, 40.3008) -> (77.8325, 46.3008) construction
  line L252 (77.8325, 46.3008) -> (80.3325, 46.3008) construction
  line L253 (80.3325, 46.3008) -> (80.3325, 40.3008) construction
  line L254 (87.8325, 48.4258) -> (87.8325, 38.1758) construction
  line L255 (75.8325, 48.4258) -> (75.8325, 38.1758) construction
  line L256 (41.6663, 38.1758) -> (24.9998, 38.1758) construction
  line L257 (24.9998, 38.1758) -> (24.9998, 48.4258) construction
  line L258 (24.9998, 48.4258) -> (41.6663, 48.4258) construction
  line L259 (41.6663, 48.4258) -> (41.6663, 38.1758) construction
  line L260 (35.833, 40.8008) -> (30.833, 40.8008) construction
  line L261 (30.833, 40.8008) -> (30.833, 45.8008) construction
  line L262 (30.833, 45.8008) -> (35.833, 45.8008) construction
  line L263 (35.833, 45.8008) -> (35.833, 40.8008) construction
  line L264 (33.333, 38.1758) -> (33.333, 48.4258) construction
  line L265 (41.6663, 43.3008) -> (24.9998, 43.3008) construction
  line L266 (30.333, 40.3008) -> (27.833, 40.3008) construction
  line L267 (27.833, 40.3008) -> (27.833, 46.3008) construction
  line L268 (27.833, 46.3008) -> (30.333, 46.3008) construction
  line L269 (30.333, 46.3008) -> (30.333, 40.3008) construction
  line L270 (37.833, 48.4258) -> (37.833, 38.1758) construction
  line L271 (25.833, 48.4258) -> (25.833, 38.1758) construction
  line L272 (74.9993, 95.9103) -> (58.3328, 95.9103) construction
  line L273 (58.3328, 95.9103) -> (58.3328, 106.1603) construction
  line L274 (58.3328, 106.1603) -> (74.9993, 106.1603) construction
  line L275 (74.9993, 106.1603) -> (74.9993, 95.9103) construction
  line L276 (69.166, 98.5353) -> (64.166, 98.5353) construction
  line L277 (64.166, 98.5353) -> (64.166, 103.5353) construction
  line L278 (64.166, 103.5353) -> (69.166, 103.5353) construction
  line L279 (69.166, 103.5353) -> (69.166, 98.5353) construction
  line L280 (66.666, 95.9103) -> (66.666, 106.1603) construction
  line L281 (74.9993, 101.0353) -> (58.3328, 101.0353) construction
  line L282 (63.666, 98.0353) -> (61.166, 98.0353) construction
  line L283 (61.166, 98.0353) -> (61.166, 104.0353) construction
  line L284 (61.166, 104.0353) -> (63.666, 104.0353) construction
  line L285 (63.666, 104.0353) -> (63.666, 98.0353) construction
  line L286 (71.166, 106.1603) -> (71.166, 95.9103) construction
  line L287 (59.166, 106.1603) -> (59.166, 95.9103) construction
  dimension "d2" = 3
  dimension "Strut_Thickness" = 2
  dimension "d12" = 2
  dimension "d13" = 2
  dimension "d14" = 2
  dimension "Strut_MateAngle" = 135
  dimension "d16" = 2
  dimension "d17" = 2
  dimension "Strut_Separation" = 0.001
  dimension "d26" = 2
  dimension "d27" = 2
  dimension "d28" = 2
  dimension "d31" = 3
  dimension "d34" = 2
  dimension "d35" = 2
  dimension "d37" = 2
  constraints: 72 point on circle, 53 tangent, 52 centre point, 45 equal radius, 36 end point, 18 coincident, 7 collinear, 6 parallel, 1 horizontal, 15 other
  measures "d2" diameter of A0
  measures "Strut_Thickness" distance between parallel lines of L2 L0
  measures "d12" distance between parallel lines of L1 L3
  measures "d13" distance between parallel lines of L1 L4
  measures "d14" distance between parallel lines of L1 L5
  measures "Strut_MateAngle" angle of L8 L6
  measures "d16" distance between parallel lines of L1 L7
  measures "d17" distance between parallel lines of L6 L9
  measures "Strut_Separation" vertical distance of L1.end L6.end
  measures "d26" distance between parallel lines of L11 L14
  measures "d27" distance between parallel lines of L11 L15
  measures "d28" distance between parallel lines of L11 L16
  measures "d31" radius of A13
  measures "d34" distance between parallel lines of L0 L12
  measures "d35" distance between parallel lines of L0 L13
  measures "d37" distance between parallel lines of L0 L17
extrude "Extrusion1" add sketch "Strut Templates" along normal blind 6 contours L1 L8 L7 A29 A28 A30 L5 A27 A26 A25 L4 A24 A23 A22 L3 A21 A19 A20 L2 A17 A13 A49 L17 A50 A51 A39 L12 A40 A35 A41 L13 A42 A34 L0 A12
equation "\"d2\" = Bolt_HoleDiameter"
equation "\"d12\" = Strut_Thickness"
equation "\"d13\" = Strut_Thickness"
equation "\"d14\" = Strut_Thickness"
equation "\"d16\" = Strut_Thickness"
equation "\"d17\" = Strut_Thickness"
equation "\"d26\" = Strut_Thickness"
equation "\"d27\" = Strut_Thickness"
equation "\"d28\" = Strut_Thickness"
equation "\"d31\" = 0.5 * Bolt_HeadDiameter"
equation "\"d34\" = Strut_Thickness"
equation "\"d35\" = Strut_Thickness"
equation "\"d37\" = Strut_Thickness"
equation "\"Bolt_HoleDiameter\" = 3"
equation "\"Bolt_HeadDiameter\" = 6"
body "Solid1"
